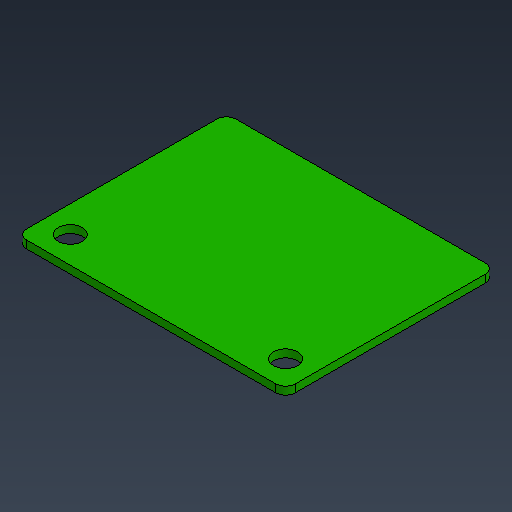
# Autodesk Inventor part: PCB_Controller
Saved by Autodesk Inventor 2026.2 (Build 302298010, 298A)
## iProperties
Created: 2026-04-05
Part Number: PCB_Controller
Material: Generic
Document SubType Name: Modeling
Designer: szymo
Density: 1 g/cm^3
Appearance: Default(1)
Mass: 0.426691 g
Surface Area: 11.6246 cm^2
Volume: 0.426691 cm^3
Author: szymo
Autodesk Inventor part; units mm, degrees
ref_plane "YZ Plane" through (0, 0, 0) normal (1, 0, 0) x (0, 1, 0)
ref_plane "XZ Plane" through (0, 0, 0) normal (0, 1, 0) x (-1, 0, 0)
ref_plane "XY Plane" through (0, 0, 0) normal (0, 0, 1) x (1, 0, 0)
ref_plane "Work Plane1" through (0.75, 1.7337, 0.1) normal (0, 0, 1) x (1, 0, 0)
sketch "Sketch1" plane through (0.75, 1.7337, 0.1) normal (0, 0, 1) x (1, 0, 0)
  line L0 (14.9531, -9.2968) -> (14.9531, -22.3927) projected
  line L1 (14.9531, -9.2968) -> (11.1531, -9.2968) projected
  line L2 (-21.9469, -9.3648) -> (-21.9469, -22.4606) projected
  line L3 (-21.9469, -22.4606) -> (-18.1469, -22.4606) projected
  line L4 (10.3531, -18.6448) -> (-17.3469, -18.6448)
  line L5 (-17.3469, -18.6448) -> (-17.3469, -17.8448)
  line L6 (-17.3469, -17.8448) -> (10.3531, -17.8448)
  line L7 (10.3531, -17.8448) -> (10.3531, -18.6448)
  line L8 (14.9531, -22.3927) -> (10.7531, -22.3927) projected
  circle A0 centre (12.7531, -12.5861) radius 2 projected
  circle A1 centre (12.7531, -12.5861) radius 2 projected
  circle A2 centre (12.7531, -19.134) radius 2 projected
  circle A3 centre (12.7531, -19.134) radius 2 projected
  line L9 (11.1531, -10.0071) -> (11.1531, -9.2968) projected
  line L10 (11.1531, -10.0071) -> (10.7531, -10.0071) projected
  line L11 (10.7531, -12.5861) -> (10.7531, -10.0071) projected
  line L12 (10.7531, -19.134) -> (10.7531, -12.5861) projected
  line L13 (10.7531, -22.3927) -> (10.7531, -19.134) projected
  line L14 (-18.1469, -21.6129) -> (-18.1469, -22.4606) projected
  line L15 (-18.1469, -21.6129) -> (-17.7469, -21.6129) projected
  line L16 (-17.7469, -9.3648) -> (-17.7469, -21.6129) projected
  line L17 (-21.9469, -9.3648) -> (-17.7469, -9.3648) projected
  circle A4 centre (-19.8469, -19.1867) radius 2 projected
  circle A5 centre (-19.8469, -12.6387) radius 2 projected
  point P0 (-0.75, -1.7337)
  point P1 (-18.5469, -9.3259)
  dimension "d2" = 0.8
  constraints: 8 end point, 2 horizontal alignment, 2 parallel, 1 horizontal, 1 perpendicular, 1 other
  measures "d2" distance between parallel lines of L6 L4
extrude "Extrusion1" add sketch "Sketch1" along normal blind 20.9 and the other way blind 0.7 contours L4 L5 L6 L7
sketch "Sketch3" plane through (-16.5969, -16.911, -0.6) normal (0, -1, 0) x (1, 0, 0)
  line L0 (27.7, 0) -> (0, 0) projected
  line L1 (27.7, 0) -> (27.7, 21.6) projected
  line L2 (0, 21.6) -> (27.7, 21.6) projected
  line L3 (0, 0) -> (0, 21.6) projected
  circle A0 centre (24.95, 18.85) radius 2.75
  circle A1 centre (2.75, 18.85) radius 2.75
  line L4 (27.7, 21.6) -> (27.7, 0)
  line L5 (0, 0) -> (0, 21.6)
  point P0 (16.5969, 0.6)
  dimension "d17" = 5.5
  dimension "d18" = 5.5
  dimension "d19" = 0
  dimension "d20" = 0
  constraints: 4 end point, 4 point on line, 4 tangent, 2 centre point, 2 perpendicular
  measures "d17" diameter of A0
  measures "d18" diameter of A1
  measures "d19" distance between parallel lines of L3 L5
  measures "d20" distance between parallel lines of L1 L4
hole "Hole1" at (8.3531, -16.911, 18.25) at (-13.8469, -16.911, 18.25) direction (0, 1, 0) diameter 2.5 end through all
fillet "Fillet1" radius 1 4 edges at (11.1031, -16.511, -0.6) (-16.5969, -16.511, -0.6) (-16.5969, -16.511, 21) (11.1031, -16.511, 21)
body "Solid1"
